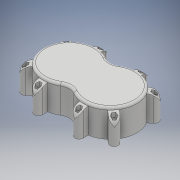
# Autodesk Inventor part: Gehaeuse_V5
Saved by Autodesk Inventor 2017 (Build 210142000, 142)
## iProperties
Created: 2019-05-23
Part Number: Gehaeuse_V5
Material: Generic
Document SubType Name: Modeling
Designer: Ole Simmering
Density: 1 g/cm^3
Appearance: Default
Author: Ole Simmering
Autodesk Inventor part; units mm, degrees
ref_plane "YZ Plane" through (0, 0, 0) normal (1, 0, 0) x (0, 1, 0)
ref_plane "XZ Plane" through (0, 0, 0) normal (0, 1, 0) x (-1, 0, 0)
ref_plane "XY Plane" through (0, 0, 0) normal (0, 0, 1) x (1, 0, 0)
sketch "Sketch1" plane through (0, 0, 0) normal (0, 0, 1) x (1, 0, 0)
  line L0 (-11.999, -0.0009) -> (209.001, -0.0009) construction
  circle A0 centre (47.001, -0.0009) radius 42.5 construction
  circle A1 centre (132.001, -0.0009) radius 42.5 construction
  circle A2 centre (47.001, -0.0009) radius 47.5625 construction
  circle A3 centre (132.001, -0.0009) radius 47.5625 construction
  arc A4 (82.1177, 32.0773) -> (-0.5615, -0.0019) centre (47.001, -0.0009) ccw
  arc A5 (179.5635, -0.0009) -> (96.8843, 32.0773) centre (132.001, -0.0009) ccw
  arc A6 (-0.5615, -0.0019) -> (82.1177, -32.079) centre (47.001, -0.0009) ccw
  arc A7 (96.8843, -32.079) -> (179.5635, -0.0009) centre (132.001, -0.0009) ccw
  arc A8 (75.7238, 47.5616) -> (-8.5615, -0.0015) centre (47.001, -0.0009) ccw
  arc A9 (187.5635, -0.0009) -> (103.2782, 47.5616) centre (132.001, -0.0009) ccw
  line L1 (47.001, 47.5616) -> (132.001, 47.5616) construction
  arc A10 (75.7238, 47.5616) -> (103.2782, 47.5616) centre (89.501, 70.3754) ccw
  arc A11 (-8.5615, -0.0015) -> (75.7238, -47.5634) centre (47.001, -0.0009) ccw
  arc A12 (103.2782, -47.5634) -> (187.5635, -0.0009) centre (132.001, -0.0009) ccw
  arc A13 (103.2782, -47.5634) -> (75.7238, -47.5634) centre (89.501, -70.3772) ccw
  arc A14 (82.1177, 32.0773) -> (96.8843, 32.0773) centre (89.501, 38.8217) ccw
  line L2 (82.1177, 32.0773) -> (96.8843, 32.0773) construction
  arc A15 (96.8843, -32.079) -> (82.1177, -32.079) centre (89.501, -38.8234) ccw
  point P0 (89.501, 21.3519)
  point P1 (46.9513, 55.5616)
  point P2 (132.0501, 55.5616)
  dimension "d5" = 221
  dimension "d6" = 85
  dimension "d7" = 85
  dimension "d8" = 85
  dimension "d9" = 95.125
  dimension "d10" = 95.125
  dimension "d12" = 8
  dimension "d20" = 10
  constraints: 36 point on circle, 16 centre point, 6 end point, 6 symmetric about line, 5 point on line, 5 tangent, 3 horizontal, 2 coincident, 2 concentric, 7 other
  measures "d5" distance of L0.start L0.end
  measures "d6" diameter of A0
  measures "d7" diameter of A1
  measures "d8" distance of A1.centre A0.centre
  measures "d9" diameter of A2
  measures "d10" diameter of A3
  measures "d12" radial gap between concentric circles of A4 A8
  measures "d20" radius of A14
extrude "Extrusion1" add sketch "Sketch1" along normal blind 50
sketch "Sketch2" plane through (0, 0, 50) normal (0, 0, 1) x (1, 0, 0)
  arc A0 (75.7238, 47.5616) -> (75.7238, -47.5634) centre (47.001, -0.0009) ccw projected
  arc A1 (75.7238, 47.5616) -> (103.2782, 47.5616) centre (89.501, 70.3754) ccw projected
  arc A2 (103.2782, -47.5634) -> (103.2782, 47.5616) centre (132.001, -0.0009) ccw projected
  arc A3 (103.2782, -47.5634) -> (75.7238, -47.5634) centre (89.501, -70.3772) ccw projected
  point P0 (0, 0)
extrude "Extrusion2" add sketch "Sketch2" along normal blind 8
fillet "Fillet1" radius 5 4 edges at (89.501, -43.7261, 58) (187.5635, -0.0009, 58) (89.501, 43.7243, 58) (-8.5615, -0.0009, 58)
sketch "Sketch8" plane through (0, 0, 0) normal (0, 0, -1) x (-1, 0, 0)
  arc A0 (-75.7238, -47.5634) -> (-75.7238, 47.5616) centre (-47.001, -0.0009) ccw construction
  arc A1 (-103.2782, 47.5616) -> (-75.7238, 47.5616) centre (-89.501, 70.3754) ccw construction
  arc A2 (-103.2782, 47.5616) -> (-103.2782, -47.5634) centre (-132.001, -0.0009) ccw construction
  arc A3 (-75.7238, -47.5634) -> (-103.2782, -47.5634) centre (-89.501, -70.3772) ccw construction
  circle A4 centre (-89.501, -0.0009) radius 110.5 construction
  line L0 (-179.6047, 28.6535) -> (-187.784, 35.5167)
  arc A5 (-176.6656, 48.7671) -> (-187.784, 35.5167) centre (-182.2248, 42.1419) ccw
  line L1 (-176.6656, 48.7671) -> (-168.4864, 41.9039)
  line L2 (-182.2248, 42.1419) -> (-174.5643, 35.714) construction
  line L3 (-273, -0.0009) -> (56, -0.0009) construction
  line L4 (-89.501, 70.3754) -> (-89.501, -70.3772) construction
  circle A6 centre (-182.2248, 42.1419) radius 4
  arc A7 (-168.4864, 41.9039) -> (-179.6047, 28.6535) centre (-132.001, -0.0009) ccw
  line L5 (0.6028, 28.6535) -> (8.782, 35.5167)
  arc A8 (8.782, 35.5167) -> (-2.3364, 48.7671) centre (3.2228, 42.1419) ccw
  line L6 (-2.3364, 48.7671) -> (-10.5156, 41.9039)
  line L7 (3.2228, 42.1419) -> (-4.4376, 35.714) construction
  circle A9 centre (3.2228, 42.1419) radius 4
  arc A10 (0.6028, 28.6535) -> (-10.5156, 41.9039) centre (-47.001, -0.0009) ccw
  line L8 (-179.6047, -28.6553) -> (-187.784, -35.5185)
  arc A11 (-187.784, -35.5185) -> (-176.6656, -48.7688) centre (-182.2248, -42.1436) ccw
  line L9 (-176.6656, -48.7688) -> (-168.4864, -41.9057)
  line L10 (-182.2248, -42.1436) -> (-174.5643, -35.7158) construction
  circle A12 centre (-182.2248, -42.1436) radius 4
  arc A13 (-179.6047, -28.6553) -> (-168.4864, -41.9057) centre (-132.001, -0.0009) ccw
  line L11 (-2.3364, -48.7688) -> (-10.5156, -41.9057)
  line L12 (3.2228, -42.1436) -> (-4.4376, -35.7158) construction
  arc A14 (-10.5156, -41.9057) -> (0.6028, -28.6553) centre (-47.001, -0.0009) ccw
  circle A15 centre (3.2228, -42.1436) radius 4
  line L13 (0.6028, -28.6553) -> (8.782, -35.5185)
  arc A16 (-2.3364, -48.7688) -> (8.782, -35.5185) centre (3.2228, -42.1436) ccw
  line L14 (-55.6496, 65.5616) -> (-55.6496, 54.8844)
  line L15 (-47.001, 65.5616) -> (-47.001, 55.5616) construction
  arc A17 (-38.3524, 54.8844) -> (-55.6496, 54.8844) centre (-47.001, -0.0009) ccw
  line L16 (-38.3524, 54.8844) -> (-38.3524, 65.5616)
  circle A18 centre (-47.001, 65.5616) radius 4
  arc A19 (-38.3524, 65.5616) -> (-55.6496, 65.5616) centre (-47.001, 65.5616) ccw
  line L17 (-38.3524, -54.8862) -> (-38.3524, -65.5634)
  arc A20 (-55.6496, -54.8862) -> (-38.3524, -54.8862) centre (-47.001, -0.0009) ccw
  line L18 (-47.001, -65.5634) -> (-47.001, -55.5634) construction
  circle A21 centre (-47.001, -65.5634) radius 4
  arc A22 (-55.6496, -65.5634) -> (-38.3524, -65.5634) centre (-47.001, -65.5634) ccw
  line L19 (-55.6496, -65.5634) -> (-55.6496, -54.8862)
  line L20 (-123.3524, 65.5616) -> (-123.3524, 54.8844)
  line L21 (-132.001, 65.5616) -> (-132.001, 55.5616) construction
  line L22 (-140.6496, 54.8844) -> (-140.6496, 65.5616)
  arc A23 (-123.3524, 65.5616) -> (-140.6496, 65.5616) centre (-132.001, 65.5616) ccw
  circle A24 centre (-132.001, 65.5616) radius 4
  arc A25 (-123.3524, 54.8844) -> (-140.6496, 54.8844) centre (-132.001, -0.0009) ccw
  line L23 (-123.3524, -65.5634) -> (-123.3524, -54.8862)
  arc A26 (-140.6496, -54.8862) -> (-123.3524, -54.8862) centre (-132.001, -0.0009) ccw
  line L24 (-132.001, -65.5634) -> (-132.001, -55.5634) construction
  line L25 (-140.6496, -54.8862) -> (-140.6496, -65.5634)
  circle A27 centre (-132.001, -65.5634) radius 4
  arc A28 (-140.6496, -65.5634) -> (-123.3524, -65.5634) centre (-132.001, -65.5634) ccw
  point P0 (0, 0)
  point P1 (-89.501, -0.0009)
  dimension "d39" = 221
  dimension "d42" = 10
  dimension "d43" = 8
  dimension "d61" = 40
  dimension "d64" = 50
  dimension "d68" = 50
  dimension "d72" = 50
  dimension "d76" = 50
  constraints: 52 end point, 35 point on circle, 25 centre point, 22 symmetric about line, 10 coincident, 3 tangent, 2 parallel, 1 horizontal, 1 line through centre, 1 midpoint, 1 point on line, 1 vertical, 69 other
  measures "d39" diameter of A4
  measures "d42" distance of L2.end L2.start
  measures "d43" diameter of A6
  measures "d61" angle of L3 L2
extrude "Extrusion4" add sketch "Sketch8" against normal blind 53
ref_plane "Work Plane1" through (174.0455, 35.2787, 53) normal (-0.6427876, 0.7660444, 0) x (0.7660444, 0.6427876, 0)
sketch "Sketch9" plane through (174.0455, 35.2787, 53) normal (-0.6427876, 0.7660444, 0) x (0.7660444, 0.6427876, 0)
  line L0 (19.3258, 53) -> (19.3258, 0) construction
  line L1 (19.3258, 0) -> (19.3258, 53) construction
  line L2 (19.3258, 18.6486) -> (26.6201, 18.6486)
  line L3 (26.6201, 18.6486) -> (26.6201, -6.0058)
  line L4 (26.6201, -6.0058) -> (0.6772, -6.0058)
  line L5 (0.6772, -6.0058) -> (0.6772, 0)
  line L6 (0, 0) -> (0.6772, 0) construction
  line L7 (0.6772, 0) -> (19.9381, 0) construction
  arc A0 (0.6772, 0) -> (19.3258, 18.6486) centre (0.6772, 18.6486) ccw
  line L8 (-54.8853, 64.8012) -> (-54.8853, -17.807) projected
  point P0 (-156.0033, 53)
  dimension "d47" = 24.6544
  dimension "d48" = 25.9429
  constraints: 12 end point, 3 point on line, 2 horizontal, 2 perpendicular, 2 point on circle, 2 tangent, 1 centre point, 1 vertical
  measures "d47" distance of L2.end L3.end
  measures "d48" distance of L3.end L4.end
revolve "Revolution1" cut sketch "Sketch9" angle 70 about axis through (132.001, -0.0009, 0) along (0, 0, 1) and the other way 150
ref_plane "Work Plane2" through (0, 0, 53) normal (0, 0, -1) x (-1, 0, 0)
sketch "Sketch11" plane through (0, 0, 53) normal (0, 0, -1) x (-1, 0, 0)
  line L0 (-187.784, 35.5167) -> (-179.6047, 28.6535) construction
  line L1 (-168.4864, 41.9039) -> (-176.6656, 48.7671) construction
  arc A0 (-168.4864, 41.9039) -> (-179.6047, 28.6535) centre (-132.001, -0.0009) ccw construction
  circle A1 centre (-182.2248, 42.1419) radius 4 construction
  line L2 (-180.2501, 36.7166) -> (-185.9359, 37.7191)
  line L3 (-185.9359, 37.7191) -> (-187.9106, 43.1444)
  line L4 (-187.9106, 43.1444) -> (-184.1994, 47.5672)
  line L5 (-184.1994, 47.5672) -> (-178.5136, 46.5646)
  line L6 (-178.5136, 46.5646) -> (-176.539, 41.1393)
  line L7 (-176.539, 41.1393) -> (-180.2501, 36.7166)
  arc A2 (-73.1391, -43.2833) -> (-105.8629, -43.2833) centre (-89.501, -70.3772) ccw projected
  arc A3 (-105.8629, 43.2815) -> (-105.8629, -43.2833) centre (-132.001, -0.0009) ccw projected
  arc A4 (-105.8629, 43.2815) -> (-73.1391, 43.2815) centre (-89.501, 70.3754) ccw projected
  arc A5 (-73.1391, -43.2833) -> (-73.1391, 43.2815) centre (-47.001, -0.0009) ccw projected
  line L8 (-89.501, 70.3754) -> (-89.501, -70.3772) construction
  arc A6 (-96.8843, 32.0773) -> (-96.8843, -32.079) centre (-132.001, -0.0009) ccw construction
  line L9 (0, 0) -> (-132.001, -0.0009) construction
  arc A7 (-176.6656, 48.7671) -> (-187.784, 35.5167) centre (-182.2248, 42.1419) ccw construction
  line L10 (-188.85, 47.7011) -> (-182.2248, 42.1419) construction
  line L11 (8.782, 35.5167) -> (0.6028, 28.6535) construction
  line L12 (-10.5156, 41.9039) -> (-2.3364, 48.7671) construction
  arc A8 (0.6028, 28.6535) -> (-10.5156, 41.9039) centre (-47.001, -0.0009) ccw construction
  circle A9 centre (3.2228, 42.1419) radius 4 construction
  line L13 (1.2481, 36.7166) -> (6.9339, 37.7191)
  line L14 (6.9339, 37.7191) -> (8.9086, 43.1444)
  line L15 (8.9086, 43.1444) -> (5.1975, 47.5672)
  line L16 (5.1975, 47.5672) -> (-0.4883, 46.5646)
  line L17 (-0.4883, 46.5646) -> (-2.463, 41.1393)
  line L18 (-2.463, 41.1393) -> (1.2481, 36.7166)
  arc A10 (8.782, 35.5167) -> (-2.3364, 48.7671) centre (3.2228, 42.1419) ccw construction
  line L19 (9.848, 47.7011) -> (3.2228, 42.1419) construction
  line L20 (-187.7835, -35.5192) -> (-179.6044, -28.6559) construction
  line L21 (-168.4858, -41.9061) -> (-176.6649, -48.7694) construction
  arc A11 (-179.6044, -28.6559) -> (-168.4858, -41.9061) centre (-132.001, -0.0009) ccw construction
  circle A12 centre (-182.2242, -42.1443) radius 4 construction
  line L22 (-180.2496, -36.719) -> (-185.9354, -37.7216)
  line L23 (-185.9354, -37.7216) -> (-187.91, -43.147)
  line L24 (-187.91, -43.147) -> (-184.1988, -47.5697)
  line L25 (-184.1988, -47.5697) -> (-178.513, -46.567)
  line L26 (-178.513, -46.567) -> (-176.5384, -41.1417)
  line L27 (-176.5384, -41.1417) -> (-180.2496, -36.719)
  arc A13 (-187.7835, -35.5192) -> (-176.6649, -48.7694) centre (-182.2242, -42.1443) ccw construction
  line L28 (-188.8493, -47.7036) -> (-182.2242, -42.1443) construction
  line L29 (-10.5151, -41.904) -> (-2.3357, -48.7671) construction
  arc A14 (-10.5151, -41.904) -> (0.6032, -28.6535) centre (-47.001, 0.0003) ccw construction
  line L30 (8.7825, -35.5166) -> (0.6032, -28.6535) construction
  circle A15 centre (3.2234, -42.1418) radius 4 construction
  line L31 (-0.4877, -46.5646) -> (-2.4624, -41.1394)
  line L32 (-2.4624, -41.1394) -> (1.2486, -36.7165)
  line L33 (1.2486, -36.7165) -> (6.9344, -37.719)
  line L34 (6.9344, -37.719) -> (8.9092, -43.1443)
  line L35 (8.9092, -43.1443) -> (5.1981, -47.5671)
  line L36 (9.8486, -47.7009) -> (3.2234, -42.1418) construction
  arc A16 (-2.3357, -48.7671) -> (8.7825, -35.5166) centre (3.2234, -42.1418) ccw construction
  line L37 (5.1981, -47.5671) -> (-0.4877, -46.5646)
  circle A17 centre (-47.001, 65.5616) radius 4 construction
  circle A18 centre (-47.001, -65.5634) radius 4 construction
  circle A19 centre (-132.001, -65.5634) radius 4 construction
  line L38 (-126.2275, -65.5634) -> (-129.1142, -70.5634)
  line L39 (-129.1142, -70.5634) -> (-134.8877, -70.5634)
  line L40 (-134.8877, -70.5634) -> (-137.7745, -65.5634)
  line L41 (-137.7745, -65.5634) -> (-134.8877, -60.5634)
  line L42 (-134.8877, -60.5634) -> (-129.1142, -60.5634)
  line L43 (-129.1142, -60.5634) -> (-126.2275, -65.5634)
  circle A20 centre (-47.001, -65.5634) radius 4 construction
  line L44 (-52.7745, -65.5634) -> (-49.8877, -70.5634)
  line L45 (-49.8877, -70.5634) -> (-44.1142, -70.5634)
  line L46 (-44.1142, -70.5634) -> (-41.2275, -65.5634)
  line L47 (-41.2275, -65.5634) -> (-44.1142, -60.5634)
  line L48 (-44.1142, -60.5634) -> (-49.8877, -60.5634)
  line L49 (-49.8877, -60.5634) -> (-52.7745, -65.5634)
  circle A21 centre (-47.0019, 65.5628) radius 4 construction
  circle A22 centre (-132.0019, 65.5616) radius 4 construction
  line L50 (-126.2284, 65.5617) -> (-129.1152, 70.5617)
  line L51 (-129.1152, 70.5617) -> (-134.8887, 70.5616)
  line L52 (-134.8887, 70.5616) -> (-137.7754, 65.5615)
  line L53 (-137.7754, 65.5615) -> (-134.8886, 60.5616)
  line L54 (-134.8886, 60.5616) -> (-129.1151, 60.5617)
  line L55 (-129.1151, 60.5617) -> (-126.2284, 65.5617)
  line L56 (-44.1151, 60.5628) -> (-49.8886, 60.5627)
  line L57 (-49.8886, 60.5627) -> (-52.7754, 65.5627)
  line L58 (-52.7754, 65.5627) -> (-49.8887, 70.5627)
  line L59 (-41.2284, 65.5628) -> (-44.1151, 60.5628)
  circle A23 centre (-47.0019, 65.5628) radius 4 construction
  line L60 (-49.8887, 70.5627) -> (-44.1152, 70.5628)
  line L61 (-44.1152, 70.5628) -> (-41.2284, 65.5628)
  point P0 (6.287, 44.713)
  point P1 (-185.2884, -44.7155)
  point P2 (6.2876, -44.7129)
  point P3 (-47.001, -69.5634)
  point P4 (-89.5019, 70.376)
  point P5 (-132.0019, 69.5616)
  point P6 (-47.0019, 69.5628)
  dimension "d52" = 10
  constraints: 120 end point, 76 symmetric about line, 12 point on circle, 8 coincident, 7 centre point, 3 vertical, 2 vertical alignment, 1 equal length, 1 horizontal, 1 perpendicular, 54 other
  measures "d52" distance between parallel lines of L4 L7
extrude "Extrusion5" cut sketch "Sketch11" along normal blind 10 contours L2 L3 L4 L5 L6 L7 | L18 L17 L16 L15 L14 L13 | L27 L26 L25 L24 L23 L22 | L31 L32 L33 L34 L35 L37 | L38 L39 L40 L41 L42 L43 | L49 L48 L47 L46 L45 L44 | L55 L54 L53 L52 L51 L50 | L56 L57 L58 L60 L61 L59
ref_plane "Work Plane3" through (4.9564, 35.2787, 0) normal (-0.6427876, -0.7660444, 0) x (0.7660444, -0.6427876, 0)
sketch "Sketch12" plane through (4.9564, 35.2787, 0) normal (-0.6427876, -0.7660444, 0) x (0.7660444, -0.6427876, 0)
  arc A0 (-0.6772, 53) -> (-19.3258, 34.3514) centre (-0.6772, 34.3514) ccw
  line L0 (-0.6772, 53) -> (-23.866, 53) construction
  line L1 (-19.3258, 34.3514) -> (-19.3258, 48.5398) construction
  ellipse E0 centre (102.7296, 53) end of major axis (102.7296, 58) minor radius 4.7312 (107.4608, 53) -> (102.7296, 58) ccw construction
  line L2 (102.7296, 58) -> (47.0868, 58) construction
  ellipse E1 centre (47.0868, 53) end of major axis (47.0868, 58) minor radius 0.7712 (47.0868, 58) -> (46.3156, 53) ccw construction
  line L3 (0, 53) -> (36.8374, 53) construction
  line L4 (0, 53) -> (0, 53) construction
  line L5 (36.8374, 53) -> (53.8717, 53) construction
  line L6 (0, 53) -> (-0.6772, 53) construction
  line L7 (-10.6772, 0) -> (-10.6772, 0) construction
  line L8 (-10.6772, 0) -> (-10.6772, 53) construction
  line L9 (-10.6772, 53) -> (-10.6772, 53) construction
  line L10 (-10.6772, 0) -> (-10.6772, 53) construction
  line L11 (-19.3258, 0) -> (-19.3258, 53) construction
  line L12 (-19.3258, 34.3514) -> (-34.3258, 34.3514)
  line L13 (-34.3258, 34.3514) -> (-34.3258, 68)
  line L14 (-34.3258, 68) -> (-0.6772, 68)
  line L15 (-0.6772, 68) -> (-0.6772, 53)
  line L16 (54.8853, -13.6) -> (54.8853, 81.6) projected
  line L17 (26.2309, 53) -> (12.9805, 53) projected
  line L18 (12.9805, 53) -> (0, 53) projected
  line L19 (53.8717, 53) -> (83.5397, 53) projected
  line L20 (83.5397, 53) -> (96.79, 53) projected
  line L21 (96.79, 53) -> (107.4608, 53) projected
  line L22 (46.3156, 53) -> (26.2309, 53) projected
  point P0 (18.8799, 0)
  point P1 (-19.3258, 16.9445)
  dimension "d56" = 15
  dimension "d57" = 15
  constraints: 12 end point, 2 horizontal, 2 perpendicular, 2 point on circle, 2 point on line, 2 tangent, 2 vertical, 1 centre point, 2 other
  measures "d56" distance of L14.end L0.start
  measures "d57" distance of L1.start L12.end
revolve "Revolution2" cut sketch "Sketch12" angle 160 about axis through (47.001, -0.0009, 0) along (0, 0, 1) and the other way 70
equation "\"d7\" = d6"
equation "\"d8\" = d6"
equation "\"d10\" = d9"
body "Solid1"
